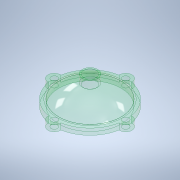
# Autodesk Inventor part: TapaS
Saved by Autodesk Inventor 2020 (Build 240168000, 168)
## iProperties
Created: 2020-10-29
Part Number: TapaS
Material: PC/ABS Plastic
Document SubType Name: Modeling
Designer: aaron
Density: 0.357273 g/cm^3
Appearance: Clear - Green 1
Author: aaron
## iProperties of the stored document _3DPrint.ipt
Created: 2020-11-03
Part Number: _3DPrint
Material: Generic
Document SubType Name: Modeling
Designer: aaron
Density: 1 g/cm^3
Appearance: Default
Author: aaron
Autodesk Inventor part; units mm, degrees
ref_plane "YZ Plane" through (0, 0, 0) normal (1, 0, 0) x (0, 1, 0)
ref_plane "XZ Plane" through (0, 0, 0) normal (0, 1, 0) x (-1, 0, 0)
sketch "Sketch1" plane through (0, 0, 0) normal (0, 1, 0) x (-1, 0, 0)
  circle A0 centre (0, 0) radius 12.5 construction
  line L0 (12.5, 0) -> (-12.5, 0) construction
  line L1 (0, -12.5) -> (0, 12.5) construction
  circle A1 centre (-11.5, 0) radius 1
  circle A2 centre (0, -11.5) radius 1
  circle A3 centre (11.5, 0) radius 1
  circle A4 centre (0, 11.5) radius 1
  circle A5 centre (0, 0) radius 10
  arc A6 (-1.9924, -11.3261) -> (1.9924, -11.3261) centre (0, -11.5) ccw
  arc A7 (-11.3261, 1.9924) -> (-11.3261, -1.9924) centre (-11.5, 0) ccw
  arc A8 (1.9924, 11.3261) -> (-1.9924, 11.3261) centre (0, 11.5) ccw
  arc A9 (11.3261, -1.9924) -> (11.3261, 1.9924) centre (11.5, 0) ccw
  arc A10 (0.9991, -11.4565) -> (11.3261, -1.9924) centre (0, 0) ccw construction
  arc A11 (1.9924, -11.3261) -> (11.3261, -1.9924) centre (0, 0) ccw
  arc A12 (11.3261, 1.9924) -> (1.9924, 11.3261) centre (0, 0) ccw construction
  arc A13 (11.3261, 1.9924) -> (1.9924, 11.3261) centre (0, 0) ccw
  arc A14 (-1.9924, 11.3261) -> (-11.3261, 1.9924) centre (0, 0) ccw construction
  arc A15 (-1.9924, 11.3261) -> (-11.3261, 1.9924) centre (0, 0) ccw
  arc A16 (-11.3261, -1.9924) -> (-1.9924, -11.3261) centre (0, 0) ccw construction
  arc A17 (-11.3261, -1.9924) -> (-1.9924, -11.3261) centre (0, 0) ccw
  line L2 (0, -10) -> (-9.6532, -10) construction
  point P0 (0, 0)
  point P1 (0, 0)
  dimension "d1" = 2
  dimension "d2" = 20
  dimension "d0" = 25
  dimension "d3" = 2
  dimension "d4" = 11.5
  dimension "d5" = 11.5
  dimension "d6" = 11.5
  dimension "d7" = 11.5
  constraints: 28 point on circle, 13 centre point, 9 coincident, 6 end point, 5 point on line, 3 equal radius, 3 horizontal, 2 horizontal alignment, 2 vertical alignment, 1 midpoint, 1 perpendicular, 14 other
  measures "d0" diameter of A0
  measures "d3" radius of A9
  measures "d4" radius of A16
  measures "d5" radius of A14
  measures "d6" radius of A12
  measures "d7" radius of A10
extrude "Extrusion1" add sketch "Sketch1" along normal blind 2
sketch "Sketch2" plane through (0, 0, 0) normal (1, 0, 0) x (0, 1, 0)
  line L0 (0, 0) -> (6.7399, 0) construction
  line L1 (2, 10.5) -> (0, 10.5) projected
  arc A0 (6.7399, 0) -> (2, 10.5) centre (-7.2601, 0) ccw
  line L2 (2, 10) -> (0, 10) projected
  arc A1 (6.2399, 0) -> (2, 10.0369) centre (-7.7601, 0) ccw
  line L3 (6.7399, 0) -> (6.7399, 0.4008)
  line L4 (2, 12.5) -> (2, 10.5) projected
  line L5 (2, 10) -> (2, 10.5)
  line L6 (0, 0) -> (-7.5749, 0) construction
  line L7 (6.7399, 0) -> (6.2399, 0)
  dimension "d10" = 14
  dimension "d11" = 0.5
  dimension "d12" = 14
  constraints: 10 end point, 4 point on circle, 3 horizontal, 3 point on line, 2 centre point, 2 vertical, 1 horizontal alignment
  measures "d10" radius of A0
  measures "d11" distance of L7.end L0.end
  measures "d12" radius of A1
revolve "Revolution1" add sketch "Sketch2" angle 360 about axis through (0, 0, 0) along (0, 1, 0)
sketch "Sketch3" plane through (0, 0, 0) normal (0, -1, 0) x (1, 0, 0)
  circle A0 centre (0, 0) radius 2
  dimension "d14" = 4
  constraints: 1 centre point, 1 coincident
  measures "d14" diameter of A0
extrude "Extrusion2" cut sketch "Sketch3" against normal up to surface
ref_plane "Work Plane1" through (0, 9, 0) normal (0, -1, 0) x (1, 0, 0)
sketch "Sketch5" plane through (0, 9, 0) normal (0, -1, 0) x (1, 0, 0)
  circle A0 centre (0, 0) radius 2
  circle A1 centre (0, 0) radius 2.5
  dimension "d20" = 5
  dimension "d21" = 4
  constraints: 2 centre point, 2 coincident
  measures "d20" diameter of A1
  measures "d21" diameter of A0
extrude "Extrusion3" add sketch "Sketch5" along normal up to surface
body "Solid1"
